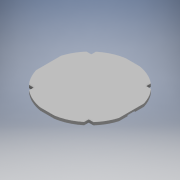
# Autodesk Inventor part: DOLNA PODSTAWA STOJAKA
Saved by Autodesk Inventor 2017 SP1 (Build 210196100, 196)
## iProperties
Created: 2020-12-25
Part Number: DOLNA PODSTAWA STOJAKA
Material: Aluminium 6061, spawane
Document SubType Name: Modeling
Designer: Napoleon
Density: 2.7 g/cm^3
Appearance: Spawane — aluminium
Mass: 51.7209 g
Surface Area: 136.896 cm^2
Volume: 19.1559 cm^3
Author: Napoleon
Autodesk Inventor part; units mm, degrees
ref_plane "YZ Plane" through (0, 0, 0) normal (1, 0, 0) x (0, 1, 0)
ref_plane "XZ Plane" through (0, 0, 0) normal (0, 1, 0) x (-1, 0, 0)
ref_plane "XY Plane" through (0, 0, 0) normal (0, 0, 1) x (1, 0, 0)
sketch "Szkic1" plane through (0, 0, 0) normal (0, 0, 1) x (1, 0, 0)
  line L0 (-33.7188, 30.3) -> (-29.425, 30.3)
  line L1 (-28.925, 30.8) -> (-28.925, 34.8858)
  line L2 (33.7188, 30.3) -> (29.425, 30.3)
  line L3 (28.925, 30.8) -> (28.925, 34.8858)
  line L4 (33.7188, -30.3) -> (29.425, -30.3)
  line L5 (28.925, -30.8) -> (28.925, -34.8858)
  line L6 (-33.7188, -30.3) -> (-29.425, -30.3)
  line L7 (-28.925, -30.8) -> (-28.925, -34.8858)
  line L8 (-7.4584, -44.8776) -> (7.4584, -44.8776)
  arc A0 (-28.7408, -35.2734) -> (-7.5413, -44.8707) centre (0, 0) ccw
  arc A1 (7.5413, -44.8707) -> (28.7408, -35.2734) centre (0, 0) ccw
  arc A2 (28.7408, 35.2734) -> (7.5413, 44.8707) centre (0, 0) ccw
  arc A3 (-7.5, 44.8776) -> (-28.7408, 35.2734) centre (0, 0) ccw
  line L9 (-43.575, 13.0209) -> (-43.575, -13.0209)
  line L10 (43.575, 13.0209) -> (43.575, -13.0209)
  arc A4 (-34.0935, 30.1311) -> (-43.5536, 13.1656) centre (0, 0) ccw
  arc A5 (-43.5536, -13.1656) -> (-34.0935, -30.1311) centre (0, 0) ccw
  arc A6 (34.0935, -30.1311) -> (43.5536, -13.1656) centre (0, 0) ccw
  arc A7 (43.5536, 13.1656) -> (34.0935, 30.1311) centre (0, 0) ccw
  line L11 (7.4584, 44.8776) -> (-7.5, 44.8776)
  arc A8 (28.925, 30.8) -> (29.425, 30.3) centre (29.425, 30.8) ccw
  arc A9 (34.0935, 30.1311) -> (33.7188, 30.3) centre (33.7188, 29.8) ccw
  arc A10 (28.925, 34.8858) -> (28.7408, 35.2734) centre (28.425, 34.8858) ccw
  arc A11 (43.575, 13.0209) -> (43.5536, 13.1656) centre (43.075, 13.0209) ccw
  arc A12 (43.5536, -13.1656) -> (43.575, -13.0209) centre (43.075, -13.0209) ccw
  arc A13 (33.7188, -30.3) -> (34.0935, -30.1311) centre (33.7188, -29.8) ccw
  arc A14 (29.425, -30.3) -> (28.925, -30.8) centre (29.425, -30.8) ccw
  arc A15 (28.7408, -35.2734) -> (28.925, -34.8858) centre (28.425, -34.8858) ccw
  arc A16 (7.4584, -44.8776) -> (7.5413, -44.8707) centre (7.4584, -44.3776) ccw
  arc A17 (-7.5413, -44.8707) -> (-7.4584, -44.8776) centre (-7.4584, -44.3776) ccw
  arc A18 (-28.925, -34.8858) -> (-28.7408, -35.2734) centre (-28.425, -34.8858) ccw
  arc A19 (-28.925, -30.8) -> (-29.425, -30.3) centre (-29.425, -30.8) ccw
  arc A20 (-34.0935, -30.1311) -> (-33.7188, -30.3) centre (-33.7188, -29.8) ccw
  arc A21 (-43.575, -13.0209) -> (-43.5536, -13.1656) centre (-43.075, -13.0209) ccw
  arc A22 (-43.5536, 13.1656) -> (-43.575, 13.0209) centre (-43.075, 13.0209) ccw
  arc A23 (-33.7188, 30.3) -> (-34.0935, 30.1311) centre (-33.7188, 29.8) ccw
  arc A24 (-29.425, 30.3) -> (-28.925, 30.8) centre (-29.425, 30.8) ccw
  arc A25 (-28.7408, 35.2734) -> (-28.925, 34.8858) centre (-28.425, 34.8858) ccw
  arc A26 (7.5413, 44.8707) -> (7.4584, 44.8776) centre (7.4584, 44.3776) ccw
  point P0 (7.5, 44.8776)
  point P1 (-28.925, 35.1226)
  point P2 (-33.9435, -30.3)
  point P3 (-33.9435, 30.3)
  point P4 (33.9435, -30.3)
  point P5 (33.9435, 30.3)
  point P6 (-28.925, 30.3)
  point P7 (28.925, 30.3)
  point P8 (28.925, 35.1226)
  point P9 (28.925, -30.3)
  point P10 (28.925, -35.1226)
  point P11 (-28.925, -30.3)
  point P12 (-28.925, -35.1226)
  point P13 (-7.5, -44.8776)
  point P14 (7.5, -44.8776)
  point P15 (-43.575, 13.0946)
  point P16 (-43.575, -13.0946)
  point P17 (43.575, 13.0946)
  point P18 (43.575, -13.0946)
  dimension "d14" = 0.5
  constraints: 69 point on circle, 38 tangent, 27 centre point, 24 end point, 24 point on line, 18 equal radius, 3 horizontal, 2 perpendicular, 1 coincident, 1 vertical
  measures "d14" radius of A8
extrude "Wyciągnięcie proste1" add sketch "Szkic1" along normal blind 3
sketch "Szkic2" plane through (0, 0, 0) normal (0, 0, -1) x (-1, 0, 0)
  line L0 (-43.575, -13.0209) -> (-43.575, 13.0209) projected
  line L1 (-43.575, -4.05) -> (-41.075, -4.05)
  line L2 (-41.075, -4.05) -> (-41.075, 4.05)
  line L3 (-41.075, 4.05) -> (-43.575, 4.05)
  line L4 (-43.575, 4.05) -> (-43.575, -4.05)
  point P0 (-42.325, 0)
  dimension "d16" = 8.1
  constraints: 8 end point, 2 parallel, 1 horizontal, 1 perpendicular
  measures "d16" distance of L2.end L1.end
extrude "Wyciągnięcie proste2" cut sketch "Szkic2" against normal blind 1
sketch "Szkic3" plane through (0, 0, 0) normal (0, 0, -1) x (-1, 0, 0)
  line L0 (-41.075, 4.05) -> (-41.075, -4.05) projected
  line L1 (-41.075, 0) -> (-31.075, 0)
  line L2 (-31.075, -3.5) -> (-31.075, 3.5)
  line L3 (-31.075, 3.5) -> (-28.075, 3.5)
  line L4 (-28.075, 3.5) -> (-28.075, -3.5)
  line L5 (-28.075, -3.5) -> (-31.075, -3.5)
  dimension "d19" = 10
  dimension "d20" = 7
  dimension "d21" = 3
  constraints: 10 end point, 2 midpoint, 2 parallel, 1 horizontal, 1 perpendicular, 1 vertical
  measures "d19" distance of L1.end L1.start
  measures "d20" distance of L2.start L2.end
  measures "d21" distance of L2.end L3.end
extrude "Wyciągnięcie proste3" add sketch "Szkic3" along normal blind 2.75
fillet "Zaokrąglenie1" radius 1 1 edges at (28.075, 0, -2.75) curvature continuous yes
